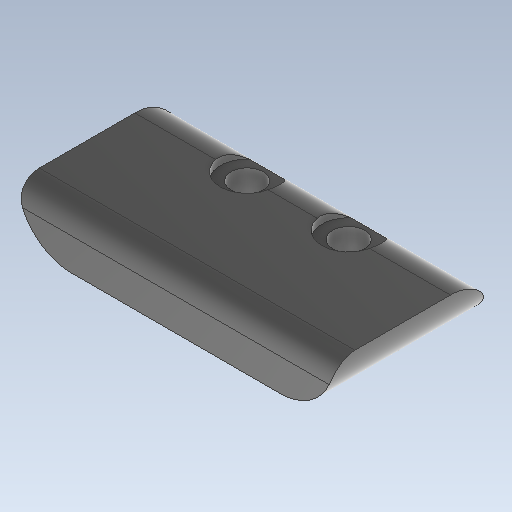
# Autodesk Inventor part: bottomclip
Saved by Autodesk Inventor 2020 (Build 240168000, 168)
## iProperties
Created: 2020-12-04
Part Number: bottomclip
Material: ABS Plastic
Document SubType Name: Modeling
Designer: Curtis
Density: 1.06 g/cm^3
Appearance: Smooth - White
Author: Curtis
Autodesk Inventor part; units mm, degrees
ref_plane "YZ Plane" through (0, 0, 0) normal (1, 0, 0) x (0, 1, 0)
ref_plane "XZ Plane" through (0, 0, 0) normal (0, 1, 0) x (-1, 0, 0)
ref_plane "XY Plane" through (0, 0, 0) normal (0, 0, 1) x (1, 0, 0)
sketch "Sketch1" plane through (0, 0, 0) normal (0, 1, 0) x (-1, 0, 0)
  line L0 (0, 0) -> (15, 0)
  line L1 (15, 0) -> (15, -29.5)
  line L2 (15, -29.5) -> (0, -29.5)
  line L3 (0, -29.5) -> (0, 0)
  dimension "d0" = 15
  dimension "d1" = 29.5
  constraints: 8 end point, 2 parallel, 1 horizontal, 1 perpendicular
  measures "d0" distance of L1.end L2.end
  measures "d1" distance of L0.end L1.end
extrude "Extrusion1" add sketch "Sketch1" along normal blind 5
fillet "Fillet1" radius 5 2 edges at (-7.5, 5, 0) (-7.5, 5, -29.5)
fillet "Fillet2" radius 4.074 1 edges at (0, 0, -14.75)
sketch "Sketch2" plane through (0, 0, 0) normal (0, -1, 0) x (1, 0, 0)
  circle A0 centre (-3.581, -10) radius 1.5
  line L0 (-15, -29.5) -> (-15, 0) projected
  line L1 (-15, -14.75) -> (-4.074, -14.75)
  line L2 (-4.074, 0) -> (-4.074, -29.5) projected
  circle A1 centre (-3.581, -19.5) radius 1.5
  line L3 (0, -27.3987) -> (0, -2.1013) projected
  point P0 (0, 0)
  dimension "d6" = 3
  dimension "d7" = 4.75
  dimension "d8" = 10.926
  dimension "d10" = 3
  dimension "d11" = 4.75
  dimension "d15" = 3.581
  dimension "d16" = 3.581
  constraints: 2 centre point, 2 end point, 2 midpoint
  measures "d6" diameter of A0
  measures "d7" distance from line of L1 A0.centre
  measures "d8" distance between parallel lines of L0 L2
  measures "d10" diameter of A1
  measures "d11" distance from line of L1 A1.centre
  measures "d15" distance from line of L3 A0.centre
  measures "d16" distance from line of L3 A1.centre
extrude "Extrusion2" cut sketch "Sketch2" against normal up to surface (5 mm away)
fillet "Fillet3" radius 1.993 1 edges at (-15, 0, -14.75)
sketch "Sketch3" plane through (0, 0, 0) normal (0, -1, 0) x (1, 0, 0)
  circle A0 centre (-3.581, -10) radius 2.5
  circle A1 centre (-3.581, -19.5) radius 2.5
  circle A2 centre (-3.581, -10) radius 1.5 projected
  circle A3 centre (-3.581, -19.5) radius 1.5 projected
  point P0 (0, 0)
  dimension "d18" = 5
  dimension "d19" = 5
  dimension "d20" = 0
  dimension "d21" = 0
  dimension "d22" = 0
  dimension "d23" = 0
  constraints: 2 centre point
  measures "d18" diameter of A0
  measures "d19" diameter of A1
  measures "d20" distance of A2.centre A0.centre
  measures "d21" distance of A2.centre A0.centre
  measures "d22" distance of A3.centre A1.centre
  measures "d23" distance of A3.centre A1.centre
extrude "Extrusion3" cut sketch "Sketch3" against normal blind 0.75
body "Solid1"
